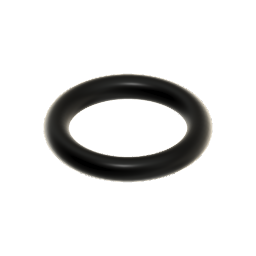
Rubber_10mm (Autodesk Fusion 360 design; units mm, degrees)
Autodesk Fusion 360 part; units mm, degrees
sketch "Sketch1" plane through (0, 0, 0) normal (0, 0, 1) x (1, 0, 0)
  circle A0 centre (0, 0) radius 5
  circle A1 centre (0, 0) radius 3.5
  dimension "d1" = 10
  dimension "d2" = 7
  constraint coincident A0.centre A1.centre
  measures "d1" diameter of A0
  measures "d2" diameter of A1
extrude "Extrude1" add sketch "Sketch1" along normal blind 1.5
fillet "Fillet1" radius 0.75 4 edges at (-4.6616, -1.8081, 1.5) (-4.6616, -1.8081, 0) (-3.2631, 1.2657, 1.5) (-3.2631, 1.2657, 0)
equation "d1 = outerDiameter"
equation "d2 = innerDiameter"
equation "d3 = height"
equation "d6 = height / 2"
equation "outerDiameter = 10 mm"
equation "innerDiameter = 7 mm"
equation "height = 1.5 mm"
named bodies: "Rubber_10mm"
